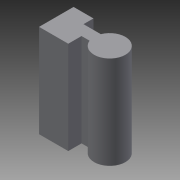
# Autodesk Inventor part: rigid connector
Saved by Autodesk Inventor 2015 (Build 190159000, 159)
## iProperties
Created: 2014-07-29
Part Number: rigid connector
Material: Generic
Document SubType Name: Modeling
Designer: Nick
Density: 1 g/cm^3
Appearance: Default
Author: Nick
Autodesk Inventor part; units mm, degrees
ref_plane "YZ Plane" through (0, 0, 0) normal (1, 0, 0) x (0, 1, 0)
ref_plane "XZ Plane" through (0, 0, 0) normal (0, 1, 0) x (-1, 0, 0)
ref_plane "XY Plane" through (0, 0, 0) normal (0, 0, 1) x (1, 0, 0)
sketch "Sketch1" plane through (0, 0, 0) normal (0, 0, 1) x (1, 0, 0)
  circle A0 centre (0, 0) radius 2.35
  line L0 (-2.1909, 0.85) -> (-4.8, 0.85)
  line L1 (-4.8, 0.85) -> (-4.8, 2.35)
  line L2 (-2.1909, -0.85) -> (-3.4, -0.85)
  line L3 (-3.4, -0.85) -> (-3.4, -2.85)
  line L4 (-3.4, -2.85) -> (-7.8, -2.85)
  line L5 (-7.8, -2.85) -> (-7.8, 2.35)
  line L6 (-7.8, 2.35) -> (-4.8, 2.35)
  dimension "d0" = 4.7
  dimension "d1" = 4.8
  dimension "d2" = 1.4
  dimension "d3" = 2
  dimension "d7" = 1.7
  dimension "d8" = 3
  dimension "d9" = 2.35
  constraints: 14 end point, 5 perpendicular, 2 point on circle, 1 centre point, 1 coincident, 1 horizontal, 1 parallel, 1 vertical alignment
  measures "d0" diameter of A0
  measures "d1" distance from line of A0.centre L1
  measures "d2" distance between parallel lines of L1 L3
  measures "d3" distance of L2.end L3.end
  measures "d7" distance between parallel lines of L2 L0
  measures "d8" distance of L5.end L1.end
  measures "d9" vertical distance of A0.centre L5.end
extrude "Extrusion1" add sketch "Sketch1" along normal blind 14
body "Solid1"
